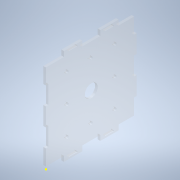
# Autodesk Inventor part: Box side 1
Saved by Autodesk Inventor 2020 (Build 240168000, 168)
## iProperties
Created: 2019-12-19
Part Number: Box side 1
Material: PMMA Plastic
Document SubType Name: Modeling
Designer: jstr255
Density: 1.188 g/cm^3
Appearance: Polycarbonate - Clear
Author: jstr255
Autodesk Inventor part; units mm, degrees
ref_plane "YZ Plane" through (0, 0, 0) normal (1, 0, 0) x (0, 1, 0)
ref_plane "XZ Plane" through (0, 0, 0) normal (0, 1, 0) x (-1, 0, 0)
ref_plane "XY Plane" through (0, 0, 0) normal (0, 0, 1) x (1, 0, 0)
sketch "Sketch1" plane through (0, 0, 0) normal (1, 0, 0) x (0, 1, 0)
  line L0 (21.2, 0) -> (21.2, -3)
  line L1 (42.4, 0) -> (42.4, -3)
  line L2 (63.6, 0) -> (63.6, -3)
  line L3 (84.8, 0) -> (84.8, -3)
  line L4 (-3, -21.2) -> (3, -21.2)
  line L5 (-3, -42.4) -> (3, -42.4)
  line L6 (-3, -63.6) -> (3, -63.6)
  line L7 (-3, -84.8) -> (3, -84.8)
  line L8 (21.2, -106) -> (21.2, -103)
  line L9 (42.4, -106) -> (42.4, -103)
  line L10 (63.6, -106) -> (63.6, -103)
  line L11 (84.8, -106) -> (84.8, -103)
  line L12 (109, -84.8) -> (103, -84.8)
  line L13 (109, -63.6) -> (103, -63.6)
  line L14 (109, -42.4) -> (103, -42.4)
  line L15 (109, -21.2) -> (103, -21.2)
  line L16 (3, -103) -> (3, -84.8)
  line L17 (3, -63.6) -> (3, -42.4)
  line L18 (3, -21.2) -> (3, -3)
  line L19 (103, -3) -> (103, -21.2)
  line L20 (103, -42.4) -> (103, -63.6)
  line L21 (103, -84.8) -> (103, -103)
  line L22 (21.2, -103) -> (3, -103)
  line L23 (84.8, -106) -> (63.6, -106)
  line L24 (42.4, -106) -> (21.2, -106)
  line L25 (103, -103) -> (84.8, -103)
  line L26 (63.6, -103) -> (42.4, -103)
  line L27 (103, -3) -> (103, 0)
  line L28 (3, -3) -> (3, 0)
  line L29 (3, 0) -> (21.2, 0)
  line L30 (21.2, -3) -> (42.4, -3)
  line L31 (63.6, -3) -> (84.8, -3)
  line L32 (42.4, 0) -> (63.6, 0)
  line L33 (84.8, 0) -> (103, 0)
  line L34 (-3, -63.6) -> (-3, -84.8)
  line L35 (-3, -21.2) -> (-3, -42.4)
  line L36 (109, -21.2) -> (109, -42.4)
  line L37 (109, -63.6) -> (109, -84.8)
  line L38 (-1, -26.8) -> (0, -26.8)
  line L39 (0, -26.8) -> (0, -36.8)
  line L40 (0, -36.8) -> (-1, -36.8)
  line L41 (-1, -36.8) -> (-1, -26.8)
  line L42 (0, -79.2) -> (-1, -79.2)
  line L43 (-1, -79.2) -> (-1, -69.2)
  line L44 (-1, -69.2) -> (0, -69.2)
  line L45 (0, -69.2) -> (0, -79.2)
  line L46 (106, -26.8) -> (107, -26.8)
  line L47 (107, -26.8) -> (107, -36.8)
  line L48 (107, -36.8) -> (106, -36.8)
  line L49 (106, -36.8) -> (106, -26.8)
  line L50 (106, -69.2) -> (105, -69.2)
  line L51 (105, -69.2) -> (105, -79.2)
  line L52 (105, -79.2) -> (106, -79.2)
  line L53 (106, -79.2) -> (106, -69.2)
  point P0 (0, 0)
  dimension "d109" = 10
  dimension "d110" = 10
  dimension "d111" = 1
  dimension "d112" = 10
  dimension "d113" = 1
  dimension "d114" = 10
  constraints: 108 end point, 37 perpendicular, 32 parallel, 9 horizontal, 8 point on line, 3 vertical, 2 collinear
  measures "d109" distance of L38.end L39.end
  measures "d110" distance of L42.end L43.end
  measures "d111" distance of L47.end L48.end
  measures "d112" distance of L46.end L47.end
  measures "d113" distance of L52.end L51.end
  measures "d114" distance of L51.end L50.end
extrude "Extrusion1" add sketch "Sketch1" along normal blind 3
sketch "Sketch3" plane through (3, 0, 0) normal (1, 0, 0) x (0, 0, -1)
  circle A0 centre (53, 53) radius 5
  point P0 (0, 0)
  dimension "d6" = 10
  constraints: 1 centre point
  measures "d6" diameter of A0
hole "Hole1" at (3, 53, -53) direction (-1, 0, 0) diameter 15 end through all
sketch "Sketch5" plane through (3, 0, 0) normal (1, 0, 0) x (0, 0, -1)
  circle A0 centre (25, 20) radius 1.5
  point P0 (0, 0)
  dimension "d45" = 3
  constraints: 1 centre point
  measures "d45" diameter of A0
hole "Hole4" at (3, 20, -25) direction (-1, 0, 0) diameter 3 end through all
sketch "Sketch6" plane through (3, 0, 0) normal (1, 0, 0) x (0, 0, -1)
  circle A0 centre (53, 20) radius 1.5
  point P0 (0, 0)
  dimension "d53" = 3
  constraints: 1 centre point
  measures "d53" diameter of A0
sketch "Sketch7" plane through (3, 0, 0) normal (1, 0, 0) x (0, 0, -1)
  point P0 (0, 0)
hole "Hole5" at (3, 20, -53) direction (-1, 0, 0) diameter 3 end through all
sketch "Sketch8" plane through (3, 0, 0) normal (1, 0, 0) x (0, 0, -1)
  circle A0 centre (81, 20) radius 1.5
  point P0 (0, 0)
  dimension "d61" = 3
  constraints: 1 centre point
  measures "d61" diameter of A0
hole "Hole6" at (3, 20, -81) direction (-1, 0, 0) diameter 3 end through all
sketch "Sketch9" plane through (3, 0, 0) normal (1, 0, 0) x (0, 0, -1)
  circle A0 centre (25, 53) radius 1.5
  point P0 (0, 0)
  dimension "d69" = 3
  constraints: 1 centre point
  measures "d69" diameter of A0
hole "Hole7" at (3, 53, -25) direction (-1, 0, 0) diameter 3 end through all
sketch "Sketch10" plane through (3, 0, 0) normal (1, 0, 0) x (0, 0, -1)
  circle A0 centre (81, 53) radius 1.5
  point P0 (0, 0)
  dimension "d77" = 3
  constraints: 1 centre point
  measures "d77" diameter of A0
hole "Hole8" at (3, 53, -81) direction (-1, 0, 0) diameter 3 end through all
sketch "Sketch11" plane through (3, 0, 0) normal (1, 0, 0) x (0, 0, -1)
  circle A0 centre (25, 86) radius 1.5
  point P0 (0, 0)
  dimension "d85" = 3
  constraints: 1 centre point
  measures "d85" diameter of A0
hole "Hole9" at (3, 86, -25) direction (-1, 0, 0) diameter 3 end through all
sketch "Sketch12" plane through (3, 0, 0) normal (1, 0, 0) x (0, 0, -1)
  circle A0 centre (53, 86) radius 1.5
  point P0 (0, 0)
  dimension "d93" = 3
  constraints: 1 centre point
  measures "d93" diameter of A0
hole "Hole10" at (3, 86, -53) direction (-1, 0, 0) diameter 3 end through all
sketch "Sketch13" plane through (3, 0, 0) normal (1, 0, 0) x (0, 0, -1)
  circle A0 centre (81, 86) radius 1.5
  point P0 (0, 0)
  dimension "d101" = 3
  constraints: 1 centre point
  measures "d101" diameter of A0
hole "Hole11" at (3, 86, -81) direction (-1, 0, 0) diameter 3 end through all
body "Solid1"
